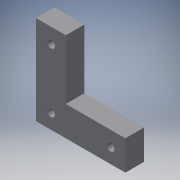
# Autodesk Inventor part: battery corner
Saved by Autodesk Inventor 2016 (Build 200138000, 138)
## iProperties
Created: 2016-02-26
Part Number: battery corner
Material: ABS Plastic
Document SubType Name: Modeling
Designer: gus
Density: 1.06 g/cm^3
Appearance: Smooth - White
Author: gus
Autodesk Inventor part; units mm, degrees
ref_plane "YZ Plane" through (0, 0, 0) normal (1, 0, 0) x (0, 1, 0)
ref_plane "XZ Plane" through (0, 0, 0) normal (0, 1, 0) x (-1, 0, 0)
ref_plane "XY Plane" through (0, 0, 0) normal (0, 0, 1) x (1, 0, 0)
sketch "Sketch1" plane through (0, 0, 0) normal (0, 0, 1) x (1, 0, 0)
  line L0 (-25.4, 50.8) -> (-25.4, -25.4)
  line L1 (-25.4, -25.4) -> (50.8, -25.4)
  line L2 (50.8, -25.4) -> (50.8, 0)
  line L3 (50.8, 0) -> (0, 0)
  line L4 (0, 0) -> (0, 50.8)
  line L5 (0, 50.8) -> (-25.4, 50.8)
  circle A0 centre (38.1, -12.7) radius 3.3734
  circle A1 centre (-12.7, -12.7) radius 3.3734
  circle A2 centre (-12.7, 38.1) radius 3.3734
  dimension "d0" = 76.2
  dimension "d1" = 76.2
  dimension "d2" = 50.8
  dimension "d3" = 25.4
  dimension "d4" = 6.7469
  dimension "d5" = 6.7469
  dimension "d6" = 6.7469
  dimension "d7" = 12.7
  dimension "d8" = 12.7
  dimension "d9" = 12.7
  dimension "d10" = 12.7
  dimension "d11" = 12.7
  dimension "d12" = 12.7
  constraints: 12 end point, 3 centre point, 3 perpendicular, 2 parallel, 1 coincident, 1 vertical
  measures "d0" distance of L0.start L0.end
  measures "d1" distance of L0.end L1.end
  measures "d2" distance of L2.end L3.end
  measures "d3" distance of L1.end L2.end
  measures "d4" diameter of A0
  measures "d5" diameter of A1
  measures "d6" diameter of A2
  measures "d7" distance from line of L0 A1.centre
  measures "d8" distance from line of L1 A0.centre
  measures "d9" distance from line of L4 A2.centre
  measures "d10" distance from line of L5 A2.centre
  measures "d11" distance from line of L1 A1.centre
  measures "d12" distance from line of L2 A0.centre
extrude "Extrusion1" add sketch "Sketch1" along normal blind 15.875
body "Solid1"
